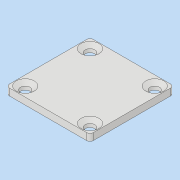
# Autodesk Inventor part: ForeAftMountPlate
Saved by Autodesk Inventor 2018 (Build 220112000, 112)
## iProperties
Created: 2019-08-15
Part Number: ForeAftMountPlate
Material: ABS Plastic
Document SubType Name: Modeling
Designer: Derek Wider
Density: 1.06 g/cm^3
Appearance: Smooth - White
Author: Derek Wider
Autodesk Inventor part; units mm, degrees
ref_plane "YZ Plane" through (0, 0, 0) normal (1, 0, 0) x (0, 1, 0)
ref_plane "XZ Plane" through (0, 0, 0) normal (0, 1, 0) x (-1, 0, 0)
ref_plane "XY Plane" through (0, 0, 0) normal (0, 0, 1) x (1, 0, 0)
sketch "Sketch1" plane through (0, 0, 0) normal (0, 1, 0) x (-1, 0, 0)
  line L0 (0, 0) -> (30.988, 0)
  line L1 (30.988, 0) -> (30.988, -30.988)
  line L2 (30.988, -30.988) -> (0, -30.988)
  line L3 (0, -30.988) -> (0, 0)
  dimension "d0" = 30.988
  dimension "d1" = 30.988
  constraints: 8 end point, 2 parallel, 1 horizontal, 1 perpendicular
  measures "d0" distance of L1.end L2.end
  measures "d1" distance of L0.end L1.end
extrude "Extrusion1" add sketch "Sketch1" along normal blind 2.54
sketch "Sketch2" plane through (0, 2.54, 0) normal (0, 1, 0) x (1, 0, 0)
  circle A0 centre (-3.556, 3.556) radius 1.778
  line L0 (0, 0) -> (0, 30.988) projected
  line L1 (-30.988, 0) -> (0, 0) projected
  circle A1 centre (-27.432, 3.556) radius 1.778
  circle A2 centre (-3.556, 27.432) radius 1.778
  circle A3 centre (-27.432, 27.432) radius 1.778
  dimension "d4" = 3.556
  dimension "d5" = 3.556
  dimension "d6" = 3.556
  dimension "d9" = 23.876
  dimension "d12" = 23.876
  constraints: 4 centre point, 1 horizontal, 1 vertical, 6 other
  measures "d4" diameter of A0
  measures "d5" distance from line of A0.centre L0
  measures "d6" distance from line of L1 A0.centre
  measures "d9" distance of A0.centre A1.centre
  measures "d12" distance of A0.centre A2.centre
extrude "Extrusion2" cut sketch "Sketch2" against normal blind 2.54
chamfer "Chamfer1" distance 1.524 distance2 1.27 1 edges at (-29.21, 2.54, -3.556) measured on face at (-11.9583, 2.54, -19.0803)
chamfer "Chamfer2" distance 1.524 distance2 1.27 1 edges at (-5.334, 2.54, -3.556) measured on face at (-18.6495, 2.54, -19.4172)
chamfer "Chamfer3" distance 1.524 distance2 1.27 1 edges at (-5.334, 2.54, -27.432) measured on face at (-18.6495, 2.54, -19.4172)
chamfer "Chamfer4" distance 1.524 distance2 1.27 1 edges at (-29.21, 2.54, -27.432) measured on face at (-19.2283, 2.54, -19.2563)
fillet "Fillet1" radius 1.27 4 edges at (0, 1.27, 0) (0, 1.27, -30.988) (-30.988, 1.27, -30.988) (-30.988, 1.27, 0)
body "Solid1"
